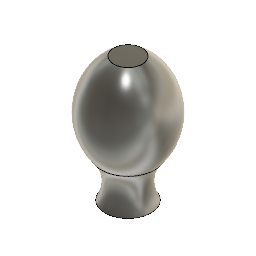
Simple_Vase (Autodesk Fusion 360 design; units mm, degrees)
Autodesk Fusion 360 part; units mm, degrees
sketch "Sketch1" plane through (0, 0, 0) normal (0, 1, 0) x (1, 0, 0)
  line L0 (-37.4232, -0.0268) -> (7.6041, -0.0268)
  arc A0 (7.6041, -0.0268) -> (15.3897, -77.353) centre (69.8425, -32.8154) ccw
  line L1 (-37.4232, -244.1309) -> (-37.4232, -0.0268)
  arc A1 (-9.5945, -244.1309) -> (15.3897, -77.353) centre (-72.7148, -149.4148) ccw
  line L2 (-9.5945, -244.1309) -> (-37.4232, -244.1309)
  line L3 (0, 0) -> (-100, 0) construction
  dimension "d1" = 113.8214
  dimension "d2" = 27.8287
  dimension "d3" = 45.0273
  dimension "d4" = 70.347
  dimension "d5" = 244.1041
  constraint perpendicular L0 L1
  constraint tangent A0 A1
  constraint coincident L3.start origin
  constraint horizontal L3
  constraint perpendicular L1 L2
  constraint parallel L0 L3
  measures "d1" radius of A1
  measures "d2" distance of L1.start A1.start
  measures "d3" distance of L0.end L0.start
  measures "d4" radius of A0
  measures "d5" vertical distance of L1.start L0.start
revolve "Revolve1" add sketch "Sketch1" angle 360 about axis through (-37.4232, 0, 244.1309) along (0, 0, -1)
shell "Shell1" thickness 4 removed faces 1 at (-28.0652, -11.7346, 0.0268)
equation "d1 = ( 70.347 * 1.618 ) * 1 mm"
equation "d3 = ( 27.829 * 1.618 ) * 1 mm"
